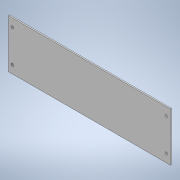
# Autodesk Inventor part: 20220624_3階部分
Saved by Autodesk Inventor 2020 (Build 240168000, 168)
## iProperties
Created: 2022-06-24
Part Number: 20220624_3階部分
Material: 一般
Document SubType Name: Modeling
Designer: Naggy
Density: 1 g/cm^3
Appearance: 既定
Author: Naggy
Autodesk Inventor part; units mm, degrees
ref_plane "YZ Plane" through (0, 0, 0) normal (1, 0, 0) x (0, 1, 0)
ref_plane "XZ Plane" through (0, 0, 0) normal (0, 1, 0) x (-1, 0, 0)
ref_plane "XY Plane" through (0, 0, 0) normal (0, 0, 1) x (1, 0, 0)
sketch "スケッチ1" plane through (0, 0, 0) normal (0, 0, 1) x (1, 0, 0)
  line L0 (-100, -30) -> (100, -30)
  line L1 (100, -30) -> (100, 30)
  line L2 (100, 30) -> (-100, 30)
  line L3 (-100, 30) -> (-100, -30)
  line L4 (-100, -30) -> (100, 30) construction
  line L5 (100, -30) -> (-100, 30) construction
  point P0 (0, 0)
  dimension "d0" = 60
  dimension "d1" = 200
  constraints: 12 end point, 2 midpoint, 2 parallel, 1 horizontal, 1 perpendicular
  measures "d0" distance between parallel lines of L0 L2
  measures "d1" distance between parallel lines of L1 L3
extrude "押し出し1" add sketch "スケッチ1" along normal blind 1.5
sketch "スケッチ2" plane through (0, 0, 1.5) normal (0, 0, 1) x (1, 0, 0)
  line L0 (-100, 30) -> (-100, -30) projected
  line L1 (100, 30) -> (-100, 30) projected
  line L2 (-100, -30) -> (100, -30) projected
  line L3 (100, -30) -> (100, 30) projected
  point P0 (0, 0)
  point P1 (-95, 20)
  point P2 (-95, -20)
  point P3 (95, 20)
  point P4 (95, -20)
  dimension "d4" = 5
  dimension "d5" = 10
  dimension "d6" = 10
  dimension "d7" = 40
  dimension "d8" = 5
  dimension "d9" = 5
  measures "d4" distance from line of point (-95, 20) L0
  measures "d5" distance from line of point (-95, 20) L1
  measures "d6" distance from line of point (-95, -20) L2
  measures "d7" distance of point (-95, -20) point (-95, 20)
  measures "d8" distance from line of point (95, 20) L3
  measures "d9" distance from line of point (95, -20) L3
hole "穴1" at (-95, 20, 1.5) at (-95, -20, 1.5) at (95, 20, 1.5) at (95, -20, 1.5) direction (0, 0, -1) diameter 3.2 depth 8.8 tip angle 118
